Autodesk Inventor part; units mm, degrees
(part 2 of 2)
equation "\"d37\" = d35"
equation "\"d38\" = d35"
equation "\"d67\" = d65"
equation "\"d68\" = d66"
equation "\"d72\" = d74"
equation "\"d73\" = d75"
equation "\"d76\" = d70"
equation "\"d77\" = d69"
body "Solid1"
